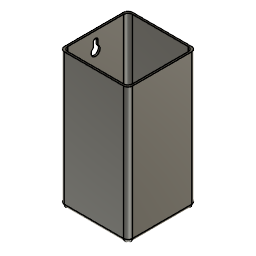
ReceiverBox (Autodesk Fusion 360 design; units mm, degrees)
Autodesk Fusion 360 part; units mm, degrees
sketch "Sketch1" plane through (0, 0, 0) normal (0, 0, 1) x (1, 0, 0)
  line L0 (0, 0) -> (76.2, 0)
  line L1 (76.2, 0) -> (76.2, 76.2)
  line L2 (76.2, 76.2) -> (0, 76.2)
  line L3 (0, 76.2) -> (0, 0)
  dimension "d1" = 76.2
  dimension "d2" = 76.2
  constraint horizontal L0
  constraint vertical L1
  constraint horizontal L2
  constraint vertical L3
  constraint coincident L0.start L3.end
  measures "d1" distance of L0.start L0.end
  measures "d2" distance of L0.start L2.end
extrude "Extrude1" add sketch "Sketch1" along normal blind 152.4
shell "Shell1" thickness 2 removed faces 1 at (25.4, 50.8, 152.4)
fillet "Fillet1" radius 5 16 edges at (2, 74.2, 77.2) (76.2, 76.2, 76.2) (76.2, 0, 76.2) (0, 0, 76.2) (38.1, 0, 0) (76.2, 38.1, 0) (38.1, 76.2, 0) (0, 76.2, 76.2) (2, 2, 77.2) (38.1, 74.2, 2) (2, 38.1, 2) (38.1, 2, 2) (74.2, 74.2, 77.2) (74.2, 38.1, 2) (74.2, 2, 77.2) (0, 38.1, 0)
sketch "Sketch2" plane through (0, 0, 0) normal (-1, 0, 0) x (0, -1, 0)
  line L0 (-5, 5) -> (-5, 152.4)
  line L1 (-5, 152.4) -> (-71.2, 152.4)
  line L2 (-71.2, 152.4) -> (-71.2, 5)
  line L3 (-71.2, 5) -> (-5, 5)
  circle A0 centre (-38.1, 132.4) radius 5
  circle A1 centre (-38.1, 142.4) radius 2.5
  line L4 (-40.6, 136.7301) -> (-40.6, 142.4)
  line L5 (-35.6, 136.7301) -> (-35.6, 142.4)
  point P0 (-38.1, 152.4)
  dimension "d8" = 10
  dimension "d9" = 5
  dimension "d10" = 10
  dimension "d11" = 10
  constraint vertical A0.centre A1.centre
  constraint midpoint L1 P0
  constraint vertical A1.centre P0
  constraint coincident A0 L4.start
  constraint coincident A1 L4.end
  constraint tangent A1 L4
  constraint coincident A0 L5.start
  constraint coincident A1 L5.end
  constraint tangent A1 L5
  constraint vertical L5
  constraint vertical L4
  measures "d8" diameter of A0
  measures "d9" diameter of A1
  measures "d10" distance of A0.centre A1.centre
  measures "d11" distance of A1.centre P0
extrude "Extrude2" cut sketch "Sketch2" against normal up to surface (2 mm away) contours A0 | A0 A1 L4 L5 | A1
